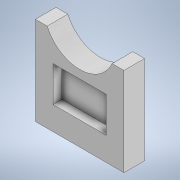
# Autodesk Inventor part: Version1
Saved by Autodesk Inventor 2021 (Build 250183000, 183)
## iProperties
Created: 2026-01-13
Part Number: Version1
Material: Generic
Document SubType Name: Modeling
Designer: Mark Bravo
Density: 1 g/cm^3
Appearance: Default
Author: Mark Bravo
Autodesk Inventor part; units mm, degrees
ref_plane "YZ Plane" through (0, 0, 0) normal (1, 0, 0) x (0, 1, 0)
ref_plane "XZ Plane" through (0, 0, 0) normal (0, 1, 0) x (-1, 0, 0)
ref_plane "XY Plane" through (0, 0, 0) normal (0, 0, 1) x (1, 0, 0)
sketch "Sketch1" plane through (0, 0, 0) normal (0, 0, 1) x (1, 0, 0)
  line L0 (-18.8022, 16.0864) -> (131.1978, 16.0864)
  line L1 (131.1978, 16.0864) -> (131.1978, -133.9136)
  line L2 (131.1978, -133.9136) -> (-18.8022, -133.9136)
  line L3 (-18.8022, -133.9136) -> (-18.8022, 16.0864)
  point P0 (0, 0)
  dimension "d0" = 150
  dimension "d1" = 150
  constraints: 8 end point, 2 parallel, 1 horizontal, 1 perpendicular
  measures "d0" distance of L0.start L0.end
  measures "d1" distance of L0.end L1.end
extrude "Extrusion1" add sketch "Sketch1" along normal blind 35
sketch "Sketch2" plane through (0, 0, 35) normal (0, 0, 1) x (1, 0, 0)
  line L0 (-18.8022, -133.9136) -> (131.1978, -133.9136) projected
  line L1 (-18.8022, 16.0864) -> (-18.8022, -133.9136) projected
  line L2 (131.1978, -133.9136) -> (131.1978, 16.0864) projected
  line L3 (-18.8022, 16.0864) -> (1.1978, 16.0864)
  line L4 (131.1978, 16.0864) -> (-18.8022, 16.0864) projected
  line L5 (131.1978, 16.0864) -> (111.1978, 16.0864)
  arc A0 (1.1978, 16.0864) -> (111.1978, 16.0864) centre (56.1978, 40.0655) ccw
  line L6 (1.1978, 16.0864) -> (111.1978, 16.0864)
  line L7 (56.1978, -93.9136) -> (-18.8022, -93.9136)
  line L8 (56.1978, -93.9136) -> (131.1978, -93.9136)
  line L9 (56.1978, -93.9136) -> (11.1978, -93.9136)
  line L10 (11.1978, -93.9136) -> (11.1978, -33.9136)
  line L11 (11.1978, -33.9136) -> (101.1978, -33.9136)
  line L12 (101.1978, -33.9136) -> (101.1978, -93.9136)
  point P0 (0, 0)
  dimension "d5" = 20
  dimension "d6" = 20
  dimension "d7" = 60
  dimension "d10" = 60
  dimension "d11" = 90
  dimension "d12" = 60
  constraints: 18 end point, 7 point on line, 3 perpendicular, 3 point on circle, 1 centre point
  measures "d5" distance of L1.start L3.end
  measures "d6" distance of L2.end L5.end
  measures "d7" radius of A0
  measures "d10" distance of L9.end L10.end
  measures "d11" distance of L10.end L11.end
  measures "d12" distance of L11.end L12.end
extrude "Extrusion2" cut sketch "Sketch2" against normal blind 35 contours L4 A0
extrude "Extrusion3" cut sketch "Sketch2" against normal blind 15 contours L10 L11 L12 L8 L7
body "Solid1"
